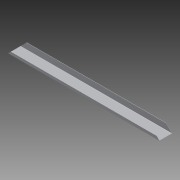
# Autodesk Inventor part: tableSide
Saved by Autodesk Inventor 2013 (Build 170138000, 138)
## iProperties
Created: 2012-10-20
Part Number: tableSide
Material: Aluminum 6061
Document SubType Name: Sheet Metal
Designer: Istvan
Density: 2.71 g/cm^3
Sheet Metal Rule: Default
Flat Pattern Width: 17.1904 cm
Flat Pattern Length: 122.396 cm
Flat Pattern Area: 2104.04 cm^2
Sheet Metal Width: 6.768 in
Sheet Metal Length: 48.188 in
Sheet Metal Area: 326.126 in^2
Mass: 1333.7 g
Surface Area: 4199.58 cm^2
Volume: 492.14 cm^3
Author: Istvan
Autodesk Inventor part; units mm, degrees
ref_plane "YZ Plane" through (0, 0, 0) normal (1, 0, 0) x (0, 1, 0)
ref_plane "XZ Plane" through (0, 0, 0) normal (0, 1, 0) x (-1, 0, 0)
ref_plane "XY Plane" through (0, 0, 0) normal (0, 0, 1) x (1, 0, 0)
sketch "Sketch1" plane through (0, 0, 0) normal (0, 1, 0) x (-1, 0, 0)
  line L0 (0, 0) -> (1249.68, 0)
  line L1 (1249.68, 0) -> (1249.68, 101.6)
  line L2 (1249.68, 101.6) -> (0, 101.6)
  line L3 (0, 101.6) -> (0, 0)
  dimension "d0" = 1249.68
  dimension "d1" = 101.6
  measures "d0" distance of L2.end L1.end
  measures "d1" distance of L1.end L0.end
extrude "Plate1" add sketch "Sketch1" against normal blind 2.3813
sketch "Sketch2" plane through (-1249.68, -2.3812, 2.3813) normal (0, 0, -1) x (-1, 0, 0)
  line L0 (-1249.68, 0) -> (0, 0)
  line L1 (0, 0) -> (0, 50.8)
  line L2 (0, 50.8) -> (-1249.68, 50.8)
  line L3 (-1249.68, 50.8) -> (-1249.68, 0)
  constraints: 6 end point, 1 horizontal, 1 perpendicular, 1 vertical
edge flange "Flange1" height 50.8 angle 90 thickness 2.3813 bend radius 2.3813 thickness toward (0, 0, -1) relief straight relief width 2.3813 relief depth 1.1906 edges at (-624.84, 0, 0) wall of the first edge with corners at (0, -2.3812, 2.3813) (-1249.68, -2.3812, 2.3813) (-1249.68, 48.4187, 2.3812) (0, 48.4187, 2.3812)
bend "Bend1"
corner "Corner1"
sketch "Sketch3" plane through (0, 0, 101.6) normal (0, 0, 1) x (1, 0, 0)
  line L0 (-1249.68, 0) -> (0, 0)
  line L1 (0, 0) -> (0, 23.0187)
  line L2 (0, 23.0187) -> (-1249.68, 23.0187)
  line L3 (-1249.68, 23.0187) -> (-1249.68, 0)
  constraints: 6 end point, 1 horizontal, 1 perpendicular, 1 vertical
edge flange "Flange2" height 25.4 angle 90 thickness 2.3813 bend radius 2.3813 thickness toward (0, 0, 1) relief straight relief width 2.3813 relief depth 1.1906 edges at (-624.84, 0, 101.6) wall of the first edge with corners at (-1249.68, 0, 101.6) (0, 0, 101.6) (0, 23.0187, 101.6) (-1249.68, 23.0187, 101.6)
bend "Bend2"
corner "Corner2"
sketch "Sketch5" plane through (-1249.68, 23.0188, 103.9813) normal (0, 0, 1) x (1, 0, 0)
  line L0 (0, -20.6375) -> (1249.68, -20.6375) projected
  line L1 (1249.68, 25.4) -> (1249.68, -20.6375) projected
  line L2 (1249.68, 25.4) -> (0, 25.4) projected
  line L3 (0, 25.4) -> (0, -20.6375) projected
  line L4 (0, -20.6375) -> (1249.68, -20.6375) projected
  line L5 (0, -25.4) -> (0, -20.6375) projected
  line L6 (1249.68, -25.4) -> (0, -25.4) projected
  line L7 (1249.68, -20.6375) -> (1249.68, -25.4) projected
  line L8 (0, -25.4) -> (50.8, 25.4)
  line L9 (1223.9625, -25.4) -> (1173.1625, 25.4)
  line L10 (0, -23.0188) -> (1249.68, -23.0188) projected
  line L11 (1249.68, -23.0188) -> (0, -23.0188) projected
  line L12 (0, -25.4) -> (0, 25.4)
  line L13 (50.8, 25.4) -> (0, 25.4)
  line L14 (1223.9625, -25.4) -> (1249.68, -25.4)
  line L15 (1249.68, -25.4) -> (1249.68, 25.4)
  line L16 (1173.1625, 25.4) -> (1249.68, 25.4)
  point P0 (1221.5812, -23.0188)
  point P1 (2.3812, -23.0188)
  dimension "d32" = 45
  dimension "d33" = 45
  dimension "d35" = 1219.2
  constraints: 14 end point, 7 point on line, 4 collinear, 1 perpendicular
  measures "d32" angle of L9 L6
  measures "d33" angle of L6 L8
  measures "d35" distance of point (1221.581, -23.019) point (2.381, -23.019)
extrude "Extrusion3" cut sketch "Sketch5" against normal through all contours L3 L2 L8 L0 | L0 L8 L10 L5 | L10 L8 L5 | L9 L2 L1 L0 | L0 L7 L10 L9 | L10 L7 L6 L9
equation "\"d3\" = BendReliefWidth"
equation "\"d4\" = BendReliefDepth"
equation "\"d5\" = MinimumRemnant"
equation "\"d6\" = BendRadius"
equation "\"d9\" = BendRadius"
equation "\"d10\" = CornerReliefSize"
equation "\"d11\" = GapSize"
equation "\"d12\" = JacobiRadiusSize"
equation "\"d13\" = BendReliefWidth"
equation "\"d14\" = BendReliefDepth"
equation "\"d15\" = MinimumRemnant"
equation "\"d16\" = BendRadius"
equation "\"d19\" = BendRadius"
equation "\"d20\" = CornerReliefSize"
equation "\"d21\" = GapSize"
equation "\"d22\" = JacobiRadiusSize"
equation "\"BendRadius\" = Thickness"
equation "\"BendReliefWidth\" = Thickness"
equation "\"BendReliefDepth\" = 0.5 * Thickness"
equation "\"CornerReliefSize\" = 4 * Thickness"
equation "\"MinimumRemnant\" = 2 * Thickness"
equation "\"TransitionRadius\" = BendRadius"
equation "\"JacobiRadiusSize\" = BendRadius"
equation "\"GapSize\" = Thickness"
equation "\"d2\" = BendRadius"
equation "\"Thickness\" = 2.38125"
body "Solid1"
